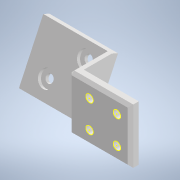
# Autodesk Inventor part: MONTURA LCD
Saved by Autodesk Inventor 2022.3 (Build 263350000, 350)
## iProperties
Created: 2022-05-17
Part Number: MONTURA LCD
Material: Genérico
Document SubType Name: Modeling
Designer: javie
Density: 1 g/cm^3
Appearance: Valor por defecto
Author: javie
Autodesk Inventor part; units mm, degrees
ref_plane "YZ Plane" through (0, 0, 0) normal (1, 0, 0) x (0, 1, 0)
ref_plane "XZ Plane" through (0, 0, 0) normal (0, 1, 0) x (-1, 0, 0)
ref_plane "XY Plane" through (0, 0, 0) normal (0, 0, 1) x (1, 0, 0)
sketch "Boceto1" plane through (0, 0, 0) normal (0, 0, 1) x (1, 0, 0)
  line L0 (30, -10) -> (-15, -10)
  line L1 (-15, -10) -> (-15, 30)
  line L2 (-15, 30) -> (30, 30)
  line L3 (30, 30) -> (30, -10)
  line L4 (-9.8, -10) -> (-4.8828, -10) projected
  line L5 (30, 24.8) -> (30, 30) projected
  line L6 (-4.8, 30) -> (-10, 30) projected
  point P0 (0, 0)
  dimension "d0" = 45
  constraints: 8 end point, 3 collinear, 2 parallel, 1 horizontal, 1 perpendicular
  measures "d0" distance of L1.end L2.end
extrude "Extrusión1" add sketch "Boceto1" along normal blind 6
sketch "Boceto2" plane through (-15, -10, 0) normal (-1, 0, 0) x (0, 0, 1)
  line L0 (-1.8126, 0.1835) -> (-18.7173, 36.4358) projected
  line L1 (0, 40) -> (-20.3793, 40)
  line L2 (-20.3793, 40) -> (-18.7173, 36.4358)
  line L3 (0, 40) -> (0, 0) projected
  line L4 (0, 0) -> (-1.8126, 0.1835)
  point P0 (0, 10)
  constraints: 6 end point, 1 collinear, 1 perpendicular
extrude "Extrusión2" add sketch "Boceto2" against normal blind 5
sketch "Boceto3" plane through (-15, -10, 6) normal (-1, 0, 0) x (0, 0, 1)
  line L0 (-7.8126, 0.1835) -> (-24.7173, 36.4358) projected
  line L1 (-8.6579, 1.9961) -> (-26.3793, 40)
  line L2 (-26.3793, 40) -> (-30.9109, 37.8869)
  line L3 (-30.9109, 37.8869) -> (-13.1894, -0.1169)
  line L4 (-13.1894, -0.1169) -> (-8.6579, 1.9961)
  point P0 (-6, 10)
  point P1 (-8.6579, 1.9961)
  point P2 (-24.7173, 36.4358)
  dimension "d5" = 2
  dimension "d6" = 5
  constraints: 8 end point, 2 parallel, 1 coincident, 1 collinear, 1 perpendicular
  measures "d5" distance of L0.start L1.start
  measures "d6" distance of L1.end L2.end
extrude "Extrusión3" add sketch "Boceto3" along normal blind 45
sketch "Boceto4" plane through (-15, -10, 6) normal (1, 0, 0) x (0, 0, -1)
  line L0 (13.1894, -0.1169) -> (8.6579, 1.9961) projected
  line L1 (30.9109, 37.8869) -> (13.1894, -0.1169) projected
  line L2 (26.3793, 40) -> (30.9109, 37.8869) projected
  line L3 (26.3793, 40) -> (8.6579, 1.9961) projected
  point P0 (6, 10)
extrude "Extrusión4" add sketch "Boceto4" along normal up to surface (5 mm away)
chamfer "Chaflán1" distance 2 angle 45 5 edges at (7.5, -10, 6) (-15, 10, 6) (-15, 30, -7.1897) (7.5, 30, 6) (30, 10, 6)
sketch "Boceto5" plane through (-15, -10, 4) normal (-1, 0, 0) x (0, 0, 1)
  line L0 (-4, 27) -> (-135.3173, 27) projected
  line L1 (-4, 33) -> (-135.3173, 33) projected
  circle A0 centre (-9, 30) radius 2.5
  line L2 (2, 2) -> (2, 38) projected
  point P0 (-4, 10)
  dimension "d14" = 5
  dimension "d15" = 6
  dimension "d16" = 3
  dimension "d17" = 11
  constraints: 1 centre point
  measures "d14" diameter of A0
  measures "d15" distance between parallel lines of L0 L1
  measures "d16" distance from line of A0.centre L1
  measures "d17" distance from line of A0.centre L2
extrude "Extrusión5" cut sketch "Boceto5" against normal blind 10
sketch "Boceto6" plane through (-60, -8.0039, -2.6579) normal (0, 0.4226183, 0.9063078) x (1, 0, 0)
  circle A0 centre (15, 12) radius 4.75 projected
  circle A1 centre (35, 32) radius 4.75 projected
  circle A2 centre (35, 32) radius 2.75
  circle A3 centre (15, 12) radius 2.75
  point P0 (60, 6.1307)
  dimension "d20" = 5.5
  dimension "d21" = 5.5
  constraints: 2 centre point, 2 coincident
  measures "d20" diameter of A2
  measures "d21" diameter of A3
extrude "Extrusión6" cut sketch "Boceto6" against normal through all contours A2 | A3
sketch "Boceto7" plane through (-60, -8.0039, -2.6579) normal (0, 0.4226183, 0.9063078) x (1, 0, 0)
  circle A0 centre (35, 32) radius 4.75 projected
  circle A1 centre (15, 12) radius 4.75 projected
  circle A2 centre (15, 12) radius 5.75
  circle A3 centre (35, 32) radius 5.75
  point P0 (60, 6.1307)
  dimension "d24" = 1
  dimension "d25" = 1
  constraints: 2 centre point
  measures "d24" radial gap between concentric circles of A1 A2
  measures "d25" radial gap between concentric circles of A0 A3
extrude "Extrusión7" cut sketch "Boceto7" against normal blind 2.5 contours A0 | A1 | A2 | A3
sketch "Boceto8" plane through (0, 0, 6) normal (0, 0, 1) x (1, 0, 0)
  circle A0 centre (20, 0) radius 2.5 projected
  circle A1 centre (20, 20) radius 2.5 projected
  circle A2 centre (0, 0) radius 2.5 projected
  circle A3 centre (0, 20) radius 2.5 projected
  circle A4 centre (20, 20) radius 2.75
  circle A5 centre (0, 20) radius 2.75
  circle A6 centre (0, 0) radius 2.75
  circle A7 centre (20, 0) radius 2.75
  dimension "d28" = 5.5
  dimension "d29" = 5.5
  dimension "d30" = 5.5
  dimension "d31" = 5.5
  constraints: 4 centre point, 4 coincident
  measures "d28" diameter of A4
  measures "d29" diameter of A5
  measures "d30" diameter of A6
  measures "d31" diameter of A7
extrude "Extrusión8" cut sketch "Boceto8" against normal through all contours A0 | A1 | A2 | A3 | A4 | A5 | A6 | A7
sketch "Boceto9" plane through (0, 0, 6) normal (0, 0, 1) x (1, 0, 0)
  circle A0 centre (20, 0) radius 2.75 projected
  circle A1 centre (0, 0) radius 2.75 projected
  circle A2 centre (0, 20) radius 2.75 projected
  circle A3 centre (20, 20) radius 2.75 projected
  circle A4 centre (20, 0) radius 5.75
  circle A5 centre (0, 0) radius 2.75 projected
  circle A6 centre (0, 0) radius 5.75
  circle A7 centre (20, 20) radius 2.75 projected
  circle A8 centre (20, 20) radius 5.75
  circle A9 centre (0, 20) radius 5.75
  dimension "d34" = 11.5
  dimension "d35" = 11.5
  dimension "d36" = 11.5
  dimension "d37" = 11.5
  constraints: 4 centre point, 4 coincident
  measures "d34" diameter of A4
  measures "d35" diameter of A6
  measures "d36" diameter of A8
  measures "d37" diameter of A9
extrude "Extrusión9" cut sketch "Boceto9" against normal blind 3
equation "\"d16\" = 0.5 * d15"
